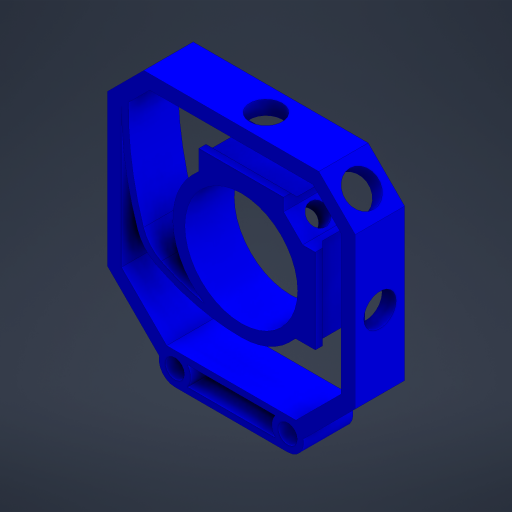
# Autodesk Inventor part: Laser Holder (USB)
Saved by Autodesk Inventor 2023.4 (Build 274418000, 418)
## iProperties
Created: 2022-07-25
Part Number: Laser Holder (USB)
Material: Generic
Document SubType Name: Modeling
Designer: xSibe
Density: 1 g/cm^3
Appearance: Plastic Blue
Author: xSibe
Autodesk Inventor part; units mm, degrees
ref_plane "YZ Plane" through (0, 0, 0) normal (1, 0, 0) x (0, 1, 0)
ref_plane "XZ Plane" through (0, 0, 0) normal (0, 1, 0) x (-1, 0, 0)
sketch "Sketch1" plane through (0, 0, 0) normal (0, 0, 1) x (1, 0, 0)
  circle A0 centre (139.6, 3.85) radius 2.8125
  circle A1 centre (159.6, 3.85) radius 2.8125
  line L0 (159.6, 1.0375) -> (139.6, 1.0375)
  line L1 (139.6, 2.145) -> (159.6, 2.145)
  line L2 (139.6, 5.555) -> (159.6, 5.555)
  line L3 (132.55, 24.9) -> (166.65, 24.9)
  line L4 (149.6, 24.9) -> (151.3678, 26.6678)
  line L5 (149.6, 24.9) -> (152.1, 24.9) construction
  circle A2 centre (151.3678, 26.6678) radius 10
  circle A3 centre (151.3678, 26.6678) radius 7.5
  circle A4 centre (151.3678, 26.6678) radius 12.125
  line L6 (151.3678, 26.6678) -> (151.3678, 38.7928)
  line L7 (151.3678, 38.7928) -> (151.3678, 37.7928)
  line L8 (143.8678, 35.7928) -> (158.8678, 35.7928)
  line L9 (158.8678, 35.7928) -> (158.8678, 39.7928)
  line L10 (158.8678, 39.7928) -> (143.8678, 39.7928)
  line L11 (143.8678, 39.7928) -> (143.8678, 35.7928)
  line L12 (143.8678, 35.7928) -> (158.8678, 39.7928) construction
  line L13 (158.8678, 35.7928) -> (143.8678, 39.7928) construction
  line L14 (151.3678, 26.6678) -> (159.9414, 35.2414)
  line L15 (159.9414, 35.2414) -> (159.4995, 34.7995)
  line L16 (162.3279, 34.0924) -> (158.7924, 37.6279)
  line L17 (158.7924, 37.6279) -> (156.6711, 35.5066)
  line L18 (156.6711, 35.5066) -> (160.2066, 31.9711)
  line L19 (160.2066, 31.9711) -> (162.3279, 34.0924)
  line L20 (162.3279, 34.0924) -> (156.6711, 35.5066) construction
  line L21 (158.7924, 37.6279) -> (160.2066, 31.9711) construction
  line L22 (162.3279, 34.0924) -> (167.3279, 34.0924) construction
  line L23 (160.4928, 19.1678) -> (160.4928, 34.1678)
  line L24 (160.4928, 34.1678) -> (164.4928, 34.1678)
  line L25 (164.4928, 34.1678) -> (164.4928, 19.1678)
  line L26 (164.4928, 19.1678) -> (160.4928, 19.1678)
  line L27 (151.3678, 38.7928) -> (151.3678, 40.7928)
  line L28 (164.4928, 26.6678) -> (166.4928, 26.6678)
  line L29 (139.3822, 5.4322) -> (159.8178, 5.4322)
  line L30 (169.0678, 14.6822) -> (169.0678, 39.3678)
  line L31 (164.0678, 44.3678) -> (135.1322, 44.3678)
  line L32 (130.1322, 39.3678) -> (130.1322, 14.6822)
  line L33 (130.1322, 5.4322) -> (169.0678, 44.3678) construction
  line L34 (169.0678, 5.4322) -> (130.1322, 44.3678) construction
  line L35 (139.3822, 5.4322) -> (130.1322, 14.6822)
  line L36 (159.8178, 5.4322) -> (169.0678, 14.6822)
  line L37 (164.0678, 44.3678) -> (169.0678, 39.3678)
  line L38 (135.1322, 44.3678) -> (130.1322, 39.3678)
  line L39 (134.0967, 46.8678) -> (127.6322, 40.4033)
  line L40 (127.6322, 40.4033) -> (127.6322, 13.6467)
  line L41 (127.6322, 13.6467) -> (138.3467, 2.9322)
  line L42 (138.3467, 2.9322) -> (160.8533, 2.9322)
  line L43 (160.8533, 2.9322) -> (171.5678, 13.6467)
  line L44 (171.5678, 13.6467) -> (171.5678, 40.4033)
  line L45 (171.5678, 40.4033) -> (165.1033, 46.8678)
  line L46 (165.1033, 46.8678) -> (134.0967, 46.8678)
  circle A5 centre (139.6, 3.85) radius 1.705
  circle A6 centre (159.6, 3.85) radius 1.705
  line L47 (151.3678, 14.5428) -> (133.8678, 14.5428)
  line L48 (133.8678, 14.5428) -> (133.8678, 19.5428)
  arc A7 (133.8678, 19.5428) -> (151.3678, 14.5428) centre (151.3678, 47.6678) ccw
  arc A8 (130.1322, 39.3678) -> (133.8678, 19.5428) centre (184.607, 39.3678) ccw
  arc A9 (131.3973, 40.6328) -> (134.8816, 20.3874) centre (184.607, 39.3678) ccw
  arc A10 (134.8816, 20.3874) -> (144.7974, 16.4773) centre (151.3678, 47.6678) ccw
  line L49 (134.8816, 20.3874) -> (134.0451, 22.7433)
  line L50 (133.8678, 19.5428) -> (133.0116, 21.8916)
  arc A11 (134.0451, 22.7433) -> (137.1762, 19.1263) centre (139.9381, 24.6809) ccw
  arc A12 (133.0116, 21.8916) -> (136.141, 18.2499) centre (139.0919, 23.9511) ccw
  line L51 (132.55, 7.7) -> (132.55, 42.1) projected
  line L52 (166.65, 7.7) -> (166.65, 42.1) projected
  circle A13 centre (139.6, 3.85) radius 1.5625 projected
  circle A14 centre (159.6, 3.85) radius 1.5625 projected
  line L53 (138.152, 6.6625) -> (161.048, 6.6625)
  point P0 (0, 0)
  point P1 (141.8368, 2.145)
  point P2 (141.8368, 5.555)
  point P3 (157.3632, 5.555)
  point P4 (157.3632, 2.145)
  point P5 (156.9415, 2.9322)
  point P6 (142.2585, 2.9322)
  point P7 (138.4142, 6.4003)
  point P8 (160.7858, 6.4003)
  point P9 (143.8678, 36.1949)
  point P10 (160.8949, 19.1678)
  point P11 (160.8949, 34.1678)
  point P12 (161.525, 33.2894)
  point P13 (157.9894, 36.825)
  point P14 (158.8678, 36.1949)
  point P15 (162.3519, 4.4308)
  point P16 (136.8481, 4.4308)
  point P17 (156.9572, 35.7928)
  point P18 (160.4928, 32.2572)
  point P19 (13.8928, 26.6678)
  point P20 (12.5533, 33.9178)
  point P21 (9.0178, 37.4533)
  point P22 (1.7678, 38.7928)
  point P23 (10.3414, 35.2414)
  point P24 (162.2525, 34.1678)
  point P25 (158.8678, 37.5525)
  point P26 (159.6, 6.6625)
  point P27 (-5.6062, 36.2928)
  point P28 (11.3928, 19.2938)
  point P29 (11.3928, 34.0417)
  point P30 (9.1417, 36.2928)
  point P31 (157.2748, 5.4322)
  point P32 (141.9252, 5.4322)
  point P33 (134.1426, 22.4687)
  dimension "d2" = 2.5
  dimension "d3" = 45
  dimension "d4" = 20
  dimension "d5" = 2.5
  dimension "d6" = 2.125
  dimension "d7" = 1
  dimension "d8" = 15
  dimension "d9" = 4
  dimension "d10" = 0.625
  dimension "d11" = 5
  dimension "d12" = 135
  dimension "d13" = 3
  dimension "d14" = 2
  dimension "d15" = 2
  dimension "d16" = 38.9355
  dimension "d17" = 38.9355
  dimension "d18" = 9.25
  dimension "d19" = 9.25
  dimension "d20" = 9.25
  dimension "d21" = 9.25
  dimension "d22" = 5
  dimension "d23" = 5
  dimension "d24" = 5
  dimension "d25" = 5
  dimension "d26" = 2.5
  dimension "d48" = 17.5
  dimension "d49" = 5
  dimension "d50" = 1.25
  dimension "d51" = 2.5
  dimension "d52" = 2.5
  dimension "d56" = 0.1425
  dimension "d57" = 0.1425
  dimension "d58" = 1.25
  dimension "d59" = 1.25
  constraints: 104 end point, 26 point on circle, 15 point on line, 12 centre point, 11 horizontal, 10 midpoint, 9 tangent, 8 parallel, 7 perpendicular, 4 symmetric about line, 3 coincident, 2 equal length, 1 vertical, 11 other
  measures "d2" distance of L4.start L4.end
  measures "d3" angle of L5 L4
  measures "d4" diameter of A2
  measures "d5" radial gap between concentric circles of A2 A3
  measures "d6" radial gap between concentric circles of A2 A4
  measures "d7" distance of L6.end L7.end
  measures "d8" distance of L10.end L9.end
  measures "d9" distance of L9.end L8.end
  measures "d10" distance of L14.end L15.end
  measures "d11" distance of L16.start L16.end
  measures "d12" angle of L22 L16
  measures "d13" distance of L17.end L16.end
  measures "d14" distance of L6.end L27.end
  measures "d15" distance of L28.start L28.end
  measures "d16" distance of L33.end L34.end
  measures "d17" distance of L34.end L33.start
  measures "d18" distance of L29.start L33.start
  measures "d19" distance of L32.end L33.start
  measures "d20" distance of L29.end L34.start
  measures "d21" distance of L30.start L34.start
  measures "d22" distance of L31.start L33.end
  measures "d23" distance of L30.end L33.end
  measures "d24" distance of L31.end L34.end
  measures "d25" distance of L32.start L34.end
  measures "d26" distance between parallel lines of L31 L46
  measures "d48" distance of L47.start L47.end
  measures "d49" distance of L47.end L48.end
  measures "d50" radial gap between concentric circles of A8 A9
  measures "d51" distance of L49.start L49.end
  measures "d52" distance of L48.end L50.end
  measures "d56" radial gap between concentric circles of A5 A13
  measures "d57" radial gap between concentric circles of A6 A14
  measures "d58" radial gap between concentric circles of A1 A14
extrude "Extrusion1" add sketch "Sketch1" along normal mid plane 8.75 contours A0 L42 A5 L29 | L29 A5 L2 A0 | A0 L1 A5 L42 | L2 A5 L35 A0 | A0 L53 A1 L2 | L29 A6 L42 A1 | A1 L2 A6 L29 | L1 A1 L0 A0 | A0 L41 A5 L1 | L42 A6 L1 A1 | A0 L35 L53 | A1 L36 A6 L2 | L1 A6 L43 A1 | L35 A5 L41 A0 | A0 L41 L51 L35 | L53 L36 A1 | L51 L41 L40 L39 L46 L45 L44 L43 L52 L36 L30 L37 L31 L38 L32 L35 | L36 L52 L43 A1 | A1 L43 A6 L36 | L51 L3 A9 A10 A4 A7 A12 A8 | A8 L38 A9 L51 | L51 A9 L3 | A11 A10 L49 | L25 L26 A4 L3 | L3 A4 L19 L16 L24 L25 | A4 L3 A2 L23 L26 | A4 L11 L8 A2 L3 | L49 A9 | A4 L26 L23 A2 L3 | L3 A2 L23 L19 A4 | L11 L10 L27 A4 | A4 L6 A2 L8 L11 | L27 L10 L9 L16 L17 A4 | A4 L17 L8 A2 L6 | L19 L23 L24 A4 | A4 L24 L16 L19 | L24 A4 L9 L16 | L17 L16 L9 A4 | A4 L9 L8 L17 | A2 L18 L19 L23 | L24 L23 L19 L18 L14 A4 | L8 L17 L18 A2 | A4 L14 L18 L17 L8 L9
sketch "Sketch2" plane through (0, 0, 0) normal (0, 0, 1) x (1, 0, 0)
  circle A0 centre (151.3678, 26.6678) radius 10 projected
  circle A1 centre (151.3678, 26.6678) radius 8.125
  point P0 (0, 0)
  dimension "d30" = 1.875
  constraints: 1 centre point
  measures "d30" radial gap between concentric circles of A0 A1
extrude "Extrusion2" [suppressed]
sketch "Sketch3" plane through (171.5678, 13.6467, -4.375) normal (1, 0, 0) x (0, 0, -1)
  line L0 (0, 5.5211) -> (-8.75, 5.5211) projected
  line L1 (0, 20.5211) -> (0, 5.5211) projected
  line L2 (-8.75, 5.5211) -> (-8.75, 20.5211) projected
  line L3 (-4.375, 20.5211) -> (-4.375, 5.5211)
  circle A0 centre (-4.375, 13.0211) radius 2.875
  line L4 (0, 20.5211) -> (-8.75, 20.5211) projected
  point P0 (-4.375, -13.6467)
  dimension "d33" = 5.75
  constraints: 3 midpoint, 2 end point, 1 centre point
  measures "d33" diameter of A0
extrude "Extrusion3" cut sketch "Sketch3" against normal up to surface (2.5 mm away) contours A0 L3 | L3 A0
sketch "Sketch4" plane through (161.8614, 34.1678, -4.375) normal (0, 1, 0) x (1, 0, 0)
  line L0 (2.6314, 0) -> (2.6314, -8.75) projected
  line L1 (0.3912, 0) -> (2.6314, 0) projected
  line L2 (2.6314, -8.75) -> (0.3912, -8.75) projected
  line L3 (2.6314, -8.75) -> (0.3912, -8.75)
  line L4 (0.3912, -8.75) -> (0.3912, -7.5)
  line L5 (0.3912, -7.5) -> (2.6314, -7.5)
  line L6 (2.6314, -7.5) -> (2.6314, -8.75)
  line L7 (2.6314, -7.5) -> (0.3912, -5.2598)
  line L8 (2.6314, -7.5) -> (5.7996, -7.5) construction
  line L9 (0.3912, -4.375) -> (2.6314, -4.375)
  line L10 (2.6314, -1.25) -> (0.3912, -3.4902)
  line L11 (1.5113, -8.75) -> (1.5113, 0)
  line L12 (0.3912, 0) -> (0.3912, -8.75) projected
  point P0 (-161.8614, -4.375)
  point P1 (2.6314, -1.25)
  point P2 (2.6314, -7.5)
  point P3 (1.5113, -2.3701)
  point P4 (1.5113, -6.3799)
  dimension "d36" = 1.25
  dimension "d37" = 135
  constraints: 18 end point, 4 midpoint, 2 horizontal, 2 parallel, 2 symmetric about line, 1 equal length, 1 perpendicular, 1 point on line
  measures "d36" distance of L2.end L4.end
  measures "d37" angle of L8 L7
extrude "Extrusion4" cut sketch "Sketch4" against normal up to surface (15 mm away) contours L0 L9 L11 L10 | L0 L7 L11 L9
ref_plane "Work Plane1" through (164.4928, 39.7928, 4.375) normal (0.7071068, -0.7071068, 0) x (0, 0, -1)
mirror "Mirror1" about plane through (164.4928, 39.7928, 4.375) normal (0.7071068, -0.7071068, 0) of "Extrusion3", "Extrusion4"
sketch "Sketch5" plane through (171.5678, 40.4033, 4.375) normal (0.7071068, 0.7071068, 0) x (0.7071068, -0.7071068, 0)
  line L0 (0, 8.75) -> (0, 0) projected
  line L1 (-9.1421, 8.75) -> (0, 8.75) projected
  line L2 (-9.1421, 8.75) -> (-9.1421, 0) projected
  line L3 (0, 0) -> (-9.1421, 0) projected
  line L4 (-6.9645, 8.75) -> (-2.1777, 8.75) projected
  line L5 (-2.1777, 0) -> (-6.9645, 0) projected
  circle A0 centre (-4.5711, 4.375) radius 1.875
  line L6 (-7.0711, 4.375) -> (-2.0711, 4.375)
  circle A1 centre (-4.5711, 4.375) radius 3
  line L7 (-6.9645, 0) -> (-6.9645, 8.75) projected
  line L8 (-2.1777, 8.75) -> (-2.1777, 0) projected
  point P0 (-92.7473, 4.375)
  dimension "d40" = 3.75
  dimension "d41" = 6
  constraints: 2 centre point, 2 end point, 1 coincident, 1 midpoint
  measures "d40" diameter of A0
  measures "d41" diameter of A1
extrude "Extrusion5" cut sketch "Sketch5" against normal up to surface (2.5 mm away) contours L8 L6 A0 L7 A1 | A1 L8 | A1 L7 L6 A0 L8 | L7 A1 | L6 A0 | A0 L6
extrude "Extrusion6" cut sketch "Sketch5" against normal up to next from surface at -10.996 contours L6 A0 | A0 L6
equation "\"d19\" = d18"
equation "\"d20\" = d18"
equation "\"d21\" = d20"
equation "\"d23\" = d22"
equation "\"d24\" = d22"
equation "\"d25\" = d24"
body "Solid1"
